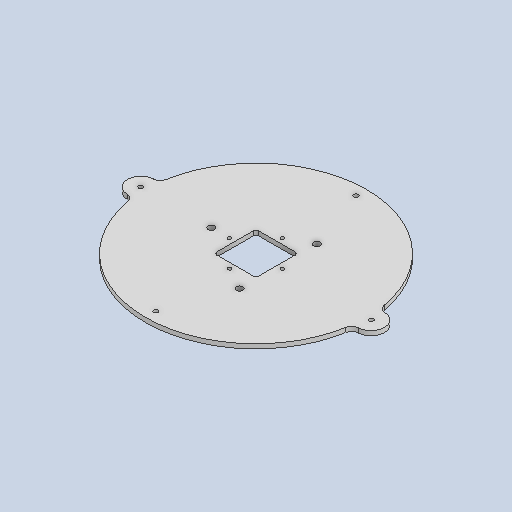
# Autodesk Inventor part: Part1
Saved by Autodesk Inventor 2025.1 (Build 291241020, 241B)
## iProperties
Created: 2024-10-16
Part Number: Part1
Material: Generic
Document SubType Name: Modeling
Designer: jdl5984
Density: 1 g/cm^3
Appearance: Default
Author: jdl5984
Autodesk Inventor part; units mm, degrees
ref_plane "YZ Plane" through (0, 0, 0) normal (1, 0, 0) x (0, 1, 0)
ref_plane "XZ Plane" through (0, 0, 0) normal (0, 1, 0) x (-1, 0, 0)
ref_plane "XY Plane" through (0, 0, 0) normal (0, 0, 1) x (1, 0, 0)
sketch "Sketch1" plane through (0, 0, 0) normal (0, 1, 0) x (-1, 0, 0)
  circle A0 centre (0, 0) radius 158.75
  line L0 (26.05, 30.05) -> (-26.05, 30.05)
  line L1 (-30.05, 26.05) -> (-30.05, -26.05)
  line L2 (-26.05, -30.05) -> (26.05, -30.05)
  line L3 (30.05, -26.05) -> (30.05, 26.05)
  arc A1 (30.05, 26.05) -> (26.05, 30.05) centre (26.05, 26.05) ccw
  arc A2 (26.05, -30.05) -> (30.05, -26.05) centre (26.05, -26.05) ccw
  arc A3 (-30.05, -26.05) -> (-26.05, -30.05) centre (-26.05, -26.05) ccw
  arc A4 (-26.05, 30.05) -> (-30.05, 26.05) centre (-26.05, 26.05) ccw
  circle A5 centre (38, 0) radius 2.5527
  circle A6 centre (0, -38) radius 2.5527
  circle A7 centre (-38, 0) radius 2.5527
  circle A8 centre (0, 38) radius 2.5527
  circle A9 centre (63.9092, 0) radius 4.7625
  circle A10 centre (-31.9546, -55.3454) radius 4.7625
  circle A11 centre (0, 0) radius 63.9092 construction
  circle A12 centre (0, 143.6497) radius 3.2067
  circle A13 centre (0, -143.6497) radius 3.2067
  line L4 (157.6029, 19.05) -> (165.227, 19.05)
  line L5 (165.227, 19.05) -> (165.227, -19.05) construction
  line L6 (165.227, -19.05) -> (157.6029, -19.05)
  line L7 (157.6029, -17.4578) -> (157.6029, 19.05) construction
  arc A14 (165.227, -19.05) -> (165.227, 19.05) centre (165.227, 0) ccw
  circle A15 centre (165.227, 0) radius 3.2067
  line L8 (0, -158.75) -> (0, 158.75) construction
  line L9 (-157.6029, 19.05) -> (-165.227, 19.05)
  line L10 (-165.227, -19.05) -> (-157.6029, -19.05)
  arc A16 (-165.227, 19.05) -> (-165.227, -19.05) centre (-165.227, 0) ccw
  circle A17 centre (-165.227, 0) radius 3.2067
  circle A18 centre (-31.9533, 55.3478) radius 4.7625
  point P0 (30.05, 30.05)
  point P1 (-30.05, 30.05)
  point P2 (30.05, -30.05)
  dimension "d0" = 317.5
  dimension "d1" = 30.05
  dimension "d2" = 60.1
  dimension "d3" = 60.1
  dimension "d4" = 30.05
  dimension "d5" = 4
  dimension "d6" = 4
  dimension "d7" = 5.1054
  dimension "d8" = 5.1054
  dimension "d9" = 5.1054
  dimension "d10" = 5.1054
  dimension "d11" = 76
  dimension "d12" = 38
  dimension "d13" = 76
  dimension "d14" = 38
  dimension "d15" = 9.525
  dimension "d17" = 110.6932
  dimension "d20" = 9.525
  dimension "d24" = 6.4135
  dimension "d25" = 6.4135
  dimension "d26" = 287.2994
  dimension "d27" = 143.6497
  dimension "d30" = 38.1
  dimension "d31" = 6.4135
  dimension "d33" = 330.454
  dimension "d38" = 110.6932
  dimension "d39" = 110.6932
  dimension "d41" = 127.8184
  constraints: 22 end point, 20 point on circle, 19 centre point, 8 tangent, 6 point on line, 6 symmetric about line, 4 coincident, 4 horizontal alignment, 4 parallel, 4 vertical alignment, 3 equal radius, 2 horizontal, 2 perpendicular, 1 midpoint, 1 vertical, 2 other
  measures "d0" diameter of A0
  measures "d1" distance from line of point (0, 0) L3
  measures "d2" distance of point (30.05, 30.05) point (-30.05, 30.05)
  measures "d3" distance of point (30.05, -30.05) point (30.05, 30.05)
  measures "d4" distance from line of point (0, 0) L2
  measures "d5" radius of A1
  measures "d6" radius of A2
  measures "d7" diameter of A5
  measures "d8" diameter of A6
  measures "d9" diameter of A7
  measures "d10" diameter of A8
  measures "d11" distance of A7.centre A5.centre
  measures "d12" distance of point (0, 0) A7.centre
  measures "d13" distance of A8.centre A6.centre
  measures "d14" distance of point (0, 0) A6.centre
  measures "d15" diameter of A9
  measures "d17" distance of A10.centre A9.centre
  measures "d20" diameter of A10
  measures "d24" diameter of A13
  measures "d25" diameter of A12
  measures "d26" distance of A13.centre A12.centre
  measures "d27" distance of A12.centre point (0, 0)
  measures "d30" distance of L4.start L6.end
  measures "d31" diameter of A15
  measures "d33" distance of A17.centre A14.centre
  measures "d38" distance of A18.centre A10.centre
  measures "d39" distance of A9.centre A18.centre
  measures "d41" diameter of A11
extrude "Extrusion1" add sketch "Sketch1" along normal blind 6.35
fillet "Fillet1" radius 10.16 4 edges at (-157.6029, 3.175, 19.05) (-157.6029, 3.175, -19.05) (157.6029, 3.175, -19.05) (157.6029, 3.175, 19.05)
equation "\"d24\" = d25"
equation "\"d25\" = d31"
equation "\"d38\" = d17"
equation "\"d39\" = d17"
body "Solid1"
